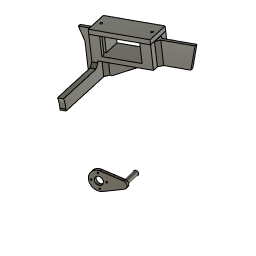
JawServoMount v26 (Autodesk Fusion 360 design; units mm, degrees)
Autodesk Fusion 360 part; units mm, degrees
sketch "BasePlate" plane through (0, 0, 0) normal (0, 0, 1) x (1, 0, 0) in component "JawServoMount"
  line L0 (0, 0) -> (105, 0)
  line L1 (105, 0) -> (105, 25) construction
  line L2 (105, 25) -> (0, 25) construction
  line L3 (0, 25) -> (0, 14)
  line L4 (0, 14) -> (-5, 0)
  line L5 (0, 0) -> (0, 14) construction
  line L6 (0, 0) -> (-5, 0)
  line L7 (105, 25) -> (112, 0)
  line L8 (112, 0) -> (105, 0)
  line L9 (0, 25) -> (0, 44)
  line L10 (0, 44) -> (24, 44)
  line L11 (24, 44) -> (64.7456, 25)
  line L12 (64.7456, 25) -> (105, 25)
  dimension "d1" = 105
  dimension "d2" = 25
  dimension "d3" = 5
  dimension "d4" = 11
  dimension "d7" = 7
  dimension "d8" = 155
  dimension "d9" = 19
  dimension "d10" = 24
  constraint horizontal L0
  constraint vertical L1
  constraint horizontal L2
  constraint vertical L3
  constraint coincident L0.start L5.start
  constraint horizontal L0.start L4.end
  constraint perpendicular L0 L5
  constraint horizontal L0.end L7.end
  constraint perpendicular L2 L9
  constraint perpendicular L9 L10
  constraint coincident L2 L11.end
  measures "d1" distance of L0.start L0.end
  measures "d2" distance of L0.start L2.end
  measures "d3" distance of L0.start L4.end
  measures "d4" distance of L2.end L3.end
  measures "d7" distance of L0.end L7.end
  measures "d8" angle of L10 L11
  measures "d9" distance of L2 L10
  measures "d10" distance of L9.end L10.end
extrude "ExtrudeBasePlate" add sketch "BasePlate" along normal blind 3.2 makes body 1 in component "JawServoMount"
sketch "Sketch1" plane through (0, 0, 0) normal (0, 0, -1) x (1, 0, 0)
  line L0 (0, -14) -> (0, -44)
  line L1 (0, -44) -> (24, -44)
  line L2 (24, -44) -> (64.7456, -25)
  line L3 (64.7456, -25) -> (105, -25)
  line L4 (105, -25) -> (112, 0)
  line L5 (112, 0) -> (-5, 0)
  line L6 (-5, 0) -> (0, -14)
sketch "CrossBeam" plane through (0, 0, 0) normal (0, 0, -1) x (1, 0, 0) in component "JawServoMount"
  line L0 (11.6, -44) -> (17.6, -44)
  line L1 (17.6, -44) -> (17.6, -31)
  line L2 (17.6, -31) -> (11.6, -31)
  line L3 (11.6, -31) -> (11.6, -44)
  line L4 (0, -44) -> (24, -44)
  line L5 (0, -14) -> (0, -44)
  point P0 (24, -44)
  dimension "d15" = 6
  dimension "d16" = 13
  dimension "d17" = 11.6
  constraint horizontal L0
  constraint vertical L1
  constraint horizontal L2
  constraint vertical L3
  constraint coincident L0.start L4
  measures "d15" distance of L0.start L0.end
  measures "d16" distance of L0.start L2.end
  measures "d17" distance of L3 L5
extrude "ExtrudeCrossBean" add sketch "CrossBeam" along normal blind 71.2 bodies 1 in component "JawServoMount"
sketch "CrossBeamEnd" plane through (17.6, 0, 0) normal (1, 0, 0) x (0, 1, 0) in component "JawServoMount"
  line L0 (31, 0) -> (31, -71.2)
  line L1 (31, -71.2) -> (44, -71.2)
  line L2 (44, -71.2) -> (44, 0)
  line L3 (31, -71.2) -> (31, -73.4)
  line L4 (42.2, -71.2) -> (38.769, -71.2766)
  line L5 (38.769, -71.2766) -> (33.7093, -71.2)
  line L6 (33.7093, -71.2) -> (31, -73.4)
  spline S0 degree 3 poles (42.2, -71.2) (38.769, -71.2766) (33.7093, -71.2) (31, -73.4) knots 0 0 0 0 1 1 1 1
  line L7 (44, 0) -> (31, 0)
  point P0 (42.2, -71.2)
  dimension "d19" = 2.2
  dimension "d20" = 1.8
  constraint coincident L0.end L1.start
  constraint perpendicular L1 L3
  constraint coincident L1 P0
  constraint coincident P0 L4.start
  constraint coincident L1 L5.end
  measures "d19" distance of L0.end L3.end
  measures "d20" distance of L1.end P0
extrude "ExtrudeCrossBeamEnd" add sketch "CrossBeamEnd" against normal up to surface (6 mm away) contours L1 L3 L6 | L1 L4 L5 S0 | L4 L5 L6 S0 bodies 1 in component "JawServoMount"
ref_plane "WorkPlane1" through (0, 20, 0) normal (0, 1, 0) x (0, 0, 1) in component "JawServoMount"
sketch "ServoBase" plane through (0, 20, 0) normal (0, 1, 0) x (1, 0, 0) in component "JawServoMount"
  line L0 (11.6, 11) -> (73.6, 11)
  line L1 (73.6, 11) -> (73.6, -16)
  line L2 (73.6, -16) -> (11.6, -16)
  line L3 (11.6, -16) -> (11.6, 11)
  line L4 (11.6, 5.6) -> (73.6, 5.6) construction
  line L5 (11.6, 3.2) -> (73.6, 3.2) construction
  line L6 (22.5, 11) -> (22.5, -16)
  line L7 (62.7, 11) -> (62.7, -16)
  line L8 (11.6, -17.2714) -> (22.5, -17.2714) construction
  line L9 (62.7, -17.2714) -> (73.6, -17.2714) construction
  line L10 (42.6, 11) -> (42.6, -16) construction
  line L11 (22.5, 3.2) -> (15.5, 3.2)
  line L12 (15.5, 5.6) -> (22.5, 7.4)
  line L13 (15.5, 5.6) -> (15.5, 3.2)
  line L14 (69.7, 5.6) -> (62.7, 7.4)
  line L15 (69.7, 5.6) -> (69.7, 3.2)
  line L16 (62.7, 3.2) -> (69.7, 3.2)
  point P0 (22.5, 5.6)
  point P1 (22.5, 7.4)
  dimension "d27" = 11.6
  dimension "d28" = 11
  dimension "d29" = 62
  dimension "d30" = 27
  dimension "d31" = 5.4
  dimension "d32" = 2.4
  dimension "d33" = 40.2
  dimension "d34" = 7
  dimension "d35" = 1.8
  constraint horizontal L0
  constraint vertical L1
  constraint horizontal L2
  constraint vertical L3
  constraint coincident L3 L4.start
  constraint coincident L1 L4.end
  constraint perpendicular L1 L4
  constraint coincident L3 L5.start
  constraint coincident L1 L5.end
  constraint perpendicular L3 L5
  constraint coincident L0 L6.start
  constraint coincident L2 L6.end
  constraint perpendicular L2 L6
  constraint coincident L0 L7.start
  constraint coincident L2 L7.end
  constraint perpendicular L2 L7
  constraint coincident L3 L8.start
  constraint coincident L6 L8.end
  constraint perpendicular L6 L8
  constraint coincident L7 L9.start
  constraint coincident L1 L9.end
  constraint perpendicular L1 L9
  constraint equal L8 L9
  constraint collinear L8 L9
  constraint midpoint L0 L10.start
  constraint midpoint L2 L10.end
  constraint coincident L5 L11.start
  constraint coincident L6 L11.start
  constraint coincident L5 L11.end
  constraint perpendicular L6 L11
  constraint coincident L4 L12.start
  constraint coincident L6 P1
  constraint perpendicular L11 L13
  constraint coincident L6 P0
  constraint coincident L4 P0
  constraint coincident P1 L12.end
  constraint symmetric L10 L11.start L16.start
  constraint symmetric L10 L11.end L15.end
  constraint symmetric L10 L12.start L14.start
  constraint symmetric L10 P1 L14.end
  measures "d27" distance of origin L3
  measures "d28" distance of origin L0
  measures "d29" distance of L1 L3
  measures "d30" distance of L0 L2
  measures "d31" distance of L0 L4
  measures "d32" distance of L4 L5
  measures "d33" distance of L6 L7
  measures "d34" distance of L6 L13
  measures "d35" distance of P0 P1
extrude "ExtrudeServoTopBottom" add sketch "ServoBase" against normal blind 20.2 contours L0 L2 L3 L6 L11 L12 L13 | L0 L1 L2 L7 L14 L15 L16 bodies 1 in component "JawServoMount"
extrude "CutServoMainPart" cut sketch "ServoBase" against normal up to surface (20.2 mm away) contours L0 L2 L6 L7 | L6 L11 L12 L13 | L7 L14 L15 L16 bodies 1 in component "JawServoMount"
extrude "ExtrudeServoBase" add sketch "ServoBase" along normal blind 5 bodies 1 in component "JawServoMount"
sketch "OtherCrossBeam" plane through (0, 0, 3.2) normal (0, 0, 1) x (-1, 0, 0) in component "JawServoMount"
  line L0 (-64.7456, -25) -> (-24, -44)
  line L1 (-24, -44) -> (0, -44)
  line L2 (0, -44) -> (0, -14)
  line L3 (0, -14) -> (5, 0)
  line L4 (-11.6, -31) -> (-11.6, -42.2)
  line L5 (-11.6, -42.2) -> (-11.6, -44)
  line L6 (-11.6, -44) -> (-17.6, -44)
  line L7 (-17.6, -44) -> (-17.6, -42.2)
  line L8 (-17.6, -42.2) -> (-17.6, -31)
  line L9 (-17.6, -31) -> (-11.6, -31)
  line L10 (-11.6, 0) -> (-11.6, -25)
  line L11 (-11.6, -25) -> (-64.7456, -25)
  line L12 (5, 0) -> (-11.6, 0)
extrude "ExtrudeOtherCrossBeam" add sketch "OtherCrossBeam" along normal blind 15.4 contours L1 L4 L5 L6 L7 L8 L9 bodies 1 in component "JawServoMount"
sketch "ServoScrewHoles" plane through (0, -0.2, 0) normal (0, -1, 0) x (1, 0, 0) in component "JawServoMount"
  line L0 (15.5, -3.2) -> (22.5, -3.2)
  line L1 (22.5, -3.2) -> (22.5, 16)
  line L2 (22.5, 16) -> (11.6, 16)
  line L3 (11.6, 16) -> (11.6, -11)
  line L4 (11.6, -11) -> (22.5, -11)
  line L5 (22.5, -11) -> (22.5, -7.4)
  line L6 (22.5, -7.4) -> (15.5, -5.6)
  line L7 (15.5, -5.6) -> (15.5, -3.2)
  line L8 (62.7, 16) -> (22.5, 16) construction
  line L9 (22.5, -11) -> (62.7, -11) construction
  line L10 (42.6, 16) -> (42.6, -11) construction
  line L11 (11.6, 16) -> (22.5, -11) construction
  line L12 (22.5, 16) -> (11.6, -11) construction
  circle A0 centre (17.05, 2.5) radius 1.4
  circle A1 centre (68.15, 2.5) radius 1.4
  dimension "d45" = 2.8
  constraint midpoint L8 L10.start
  constraint midpoint L9 L10.end
  constraint coincident L2.end L3.start
  constraint coincident L4.end L5.start
  constraint coincident L1.end L2.start
  constraint coincident L3.end L4.start
  constraint midpoint L11 A0.centre
  constraint symmetric L10 A0 A1
  measures "d45" diameter of A0
sketch "JoinCrossBeamToServoHolder" plane through (0, 31, 0) normal (0, -1, 0) x (1, 0, 0) in component "JawServoMount"
  line L0 (17.6, 0) -> (11.6, 0)
  line L1 (11.6, 0) -> (11.6, -73.4)
  line L2 (11.6, -73.4) -> (17.6, -73.4)
  line L3 (17.6, -73.4) -> (17.6, 0)
  line L4 (17.6, -11) -> (11.6, -11)
  line L5 (11.6, -11) -> (11.6, 16)
  line L6 (11.6, 16) -> (17.6, 16)
  line L7 (17.6, 16) -> (17.6, -11)
  point P0 (11.6, 16)
  constraint horizontal L4
  constraint vertical L5
  constraint horizontal L6
  constraint vertical L7
  constraint coincident P0 L5.end
  constraint coincident L3 L4.start
extrude "Extrude10" add sketch "JoinCrossBeamToServoHolder" along normal up to surface (6 mm away) contours L0 L1 L3 L4 L5 L7 | L0 L5 L6 L7 bodies 1 in component "JawServoMount"
chamfer "Chamfer3" distance 4 angle 45 9 edges at (11.6, 22, 0) (73.6, 12.5, 0) (73.6, 12.5, 3.2) (11.6, 22, 3.2) (41.1728, 25, 0) (41.1728, 25, 3.2) (17.6, 34.5, 0) (17.6, 34.5, 3.2) (14.6, 31, -11) on bodies 1 in component "JawServoMount"
chamfer "Chamfer3" distance 2.6 angle 45 1 edges at (14.6, 31, 16) on bodies 1 in component "JawServoMount"
sketch "Base" plane through (0, -0.2, 0) normal (0, -1, 0) x (1, 0, 0) in component "ServoLid"
  line L0 (62.7, -7.4) -> (62.7, -11)
  line L1 (62.7, -11) -> (73.6, -11)
  line L2 (73.6, -11) -> (73.6, 16)
  line L3 (73.6, 16) -> (62.7, 16)
  line L4 (62.7, 16) -> (62.7, -3.2)
  line L5 (62.7, -3.2) -> (69.7, -3.2)
  line L6 (69.7, -3.2) -> (69.7, -5.6)
  line L7 (69.7, -5.6) -> (62.7, -7.4)
  line L8 (73.6, 16) -> (11.6, 16)
  line L9 (11.6, 16) -> (11.6, -11)
  line L10 (11.6, -11) -> (73.6, -11)
  line L11 (73.6, -11) -> (73.6, 16)
  point P0 (11.6, -11)
  constraint horizontal L8
  constraint vertical L9
  constraint horizontal L10
  constraint vertical L11
  constraint coincident L2.end L3.start
extrude "ExtrudePlate" add sketch "Base" along normal blind 5 separate body makes body 2 in component "ServoLid"
extrude "CutScrewHoles" cut sketch "ServoScrewHoles" along normal blind -10 and the other way up to surface (-5 mm away) contours A0 | A1 bodies 1 in component "JawServoMount"
extrude "Extrude2" cut sketch "ServoScrewHoles" along normal blind -10 and the other way up to surface (-5 mm away) contours A0 | A1 bodies 2 in component "ServoLid"
sketch "Base (2)" plane through (0, 0, 0) normal (0, 0, 1) x (1, 0, 0) in component "ServoArm"
  circle A0 centre (0, 150) radius 10.4
  circle A1 centre (0, 150) radius 4.5
  circle A2 centre (24, 150) radius 4.2
  line L0 (2.6867, 160.047) -> (25.085, 154.0574)
  line L1 (2.6867, 139.953) -> (25.085, 145.9426)
  point P0 (0, 150)
  dimension "d61" = 150
  dimension "d62" = 20.8
  dimension "d63" = 9
  dimension "d72" = 8.4
  dimension "d73" = 24
  constraint vertical origin A0.centre
  constraint coincident P0 A0.centre
  constraint horizontal P0 A2.centre
  constraint coincident A0 L0.start
  constraint coincident A2 L0.end
  constraint tangent A2 L0
  constraint coincident A0 L1.start
  constraint coincident A2 L1.end
  constraint tangent A2 L1
  constraint tangent A0 L0
  constraint tangent A0 L1
  measures "d61" distance of origin A0.centre
  measures "d62" diameter of A0
  measures "d63" diameter of A1
  measures "d72" diameter of A2
  measures "d73" distance of P0 A2.centre
extrude "ExtrudeBase" add sketch "Base (2)" against normal blind 3.2 separate body makes body 3 in component "ServoArm"
sketch "ScrewHoles" plane through (0, 0, -3.2) normal (0, 0, -1) x (1, 0, 0) in component "ServoArm"
  circle A0 centre (0, -150) radius 4.5
  circle A1 centre (0, -142.25) radius 0.8
  circle A2 centre (-7.75, -150) radius 0.8
  circle A3 centre (0, -157.75) radius 0.8
  circle A4 centre (7.75, -150) radius 0.8
  arc A5 (2.6867, -139.953) -> (2.6867, -160.047) centre (0, -150) ccw
  line L0 (2.6867, -160.047) -> (25.085, -154.0574)
  arc A6 (25.085, -154.0574) -> (25.085, -145.9426) centre (24, -150) ccw
  line L1 (25.085, -145.9426) -> (2.6867, -139.953)
  point P0 (0, -142.25)
  point P1 (0, -150)
  dimension "d66" = 7.75
  dimension "d67" = 1.6
  dimension "d69" = 360
  constraint coincident P0 A1.centre
  constraint vertical A0.centre P0
  measures "d66" distance of A0.centre P0
  measures "d67" diameter of A1
extrude "ExtrudeSmallScrewHoles" cut sketch "ScrewHoles" against normal up to surface (3.2 mm away) contours A1 | A2 | A3 | A4 bodies 3 in component "ServoArm"
sketch "Pin" plane through (0, 0, 0) normal (0, 0, 1) x (1, 0, 0) in component "ServoArm"
  circle A0 centre (24, 150) radius 2.8
  point P0 (24, 150)
  dimension "d74" = 5.6
  constraint coincident P0 A0.centre
  measures "d74" diameter of A0
extrude "ExtrudePin" add sketch "Pin" along normal blind 20 bodies 3 in component "ServoArm"
chamfer "Chamfer1" distance 1.4 angle 45 1 edges at (21.3895, 151.0125, 0) on bodies 3 in component "ServoArm"
component "JawServoMount" placed x (1, 0, 0) y (0, 1, 0) z (0, 0, 1) at (0, 0, 0)
component "ServoLid" placed x (1, 0, 0) y (0, 1, 0) z (0, 0, 1) at (0, 0, 0)
component "ServoArm" placed x (1, 0, 0) y (0, 1, 0) z (0, 0, 1) at (0, 0, 0)
equation "servo_offset_down = 20 mm"
equation "servo_offset_back = 11.6 mm"
equation "servo_offset_left = 11 mm"
equation "d26 = servo_offset_down"
equation "d27 = servo_offset_back"
equation "d28 = servo_offset_left"
named bodies: "JawServoMount", "ServoLid", "ServoArm"
